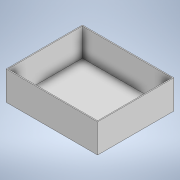
# Autodesk Inventor part: Lower Chassis
Saved by Autodesk Inventor 2020 (Build 240168000, 168)
## iProperties
Created: 2021-12-06
Part Number: Lower Chassis
Material: Generic
Document SubType Name: Modeling
Designer: dbsummers42
Density: 1 g/cm^3
Appearance: Default
Author: dbsummers42
Autodesk Inventor part; units mm, degrees
ref_plane "YZ Plane" through (0, 0, 0) normal (1, 0, 0) x (0, 1, 0)
ref_plane "XZ Plane" through (0, 0, 0) normal (0, 1, 0) x (-1, 0, 0)
ref_plane "XY Plane" through (0, 0, 0) normal (0, 0, 1) x (1, 0, 0)
sketch "Sketch1" plane through (0, 0, 0) normal (0, 1, 0) x (-1, 0, 0)
  line L0 (0, 0) -> (304.8, 0)
  line L1 (304.8, 0) -> (304.8, 254)
  line L2 (304.8, 254) -> (0, 254)
  line L3 (0, 254) -> (0, 0)
  line L4 (301.625, 250.825) -> (301.625, 3.175)
  line L5 (301.625, 3.175) -> (3.175, 3.175)
  line L6 (3.175, 3.175) -> (3.175, 250.825)
  line L7 (3.175, 250.825) -> (301.625, 250.825)
  dimension "d0" = 304.8
  dimension "d1" = 254
  dimension "d21" = 3.175
  constraints: 16 end point, 4 parallel, 2 perpendicular, 1 horizontal, 3 other
  measures "d0" distance of L2.end L1.end
  measures "d1" distance of L1.end L0.end
  measures "d21" distance between parallel lines of L1 L4
extrude "Extrusion1" add sketch "Sketch1" along normal blind 92.71
sketch "Sketch5" plane through (0, 0, 0) normal (0, -1, 0) x (1, 0, 0)
  line L0 (0, 0) -> (-304.8, 0)
  line L1 (-304.8, 0) -> (-304.8, 254)
  line L2 (-304.8, 254) -> (0, 254)
  line L3 (0, 254) -> (0, 0)
  dimension "d22" = 304.8
  dimension "d23" = 254
  constraints: 8 end point, 2 parallel, 1 horizontal, 1 perpendicular
  measures "d22" distance of L1.end L2.end
  measures "d23" distance of L0.end L1.end
extrude "Extrusion4" add sketch "Sketch5" along normal blind 3.175
body "Solid1"
